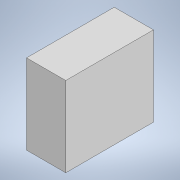
# Autodesk Inventor part: Akkuboxdummy
Saved by Autodesk Inventor 2020 (Build 240168000, 168)
## iProperties
Created: 2020-05-28
Part Number: Akkuboxdummy
Material: Generisch
Document SubType Name: Modeling
Designer: Chris
Density: 1 g/cm^3
Appearance: Vorgabe
Author: Chris
Autodesk Inventor part; units mm, degrees
ref_plane "YZ Plane" through (0, 0, 0) normal (1, 0, 0) x (0, 1, 0)
ref_plane "XZ Plane" through (0, 0, 0) normal (0, 1, 0) x (-1, 0, 0)
ref_plane "XY Plane" through (0, 0, 0) normal (0, 0, 1) x (1, 0, 0)
sketch "Skizze1" plane through (0, 0, 0) normal (0, 1, 0) x (-1, 0, 0)
  line L0 (0, 0) -> (-152, 0)
  line L1 (-152, 0) -> (-152, -340)
  line L2 (-152, -340) -> (0, -340)
  line L3 (0, -340) -> (0, 0)
  dimension "d0" = 152
  dimension "d1" = 340
  constraints: 8 end point, 2 parallel, 1 horizontal, 1 perpendicular
  measures "d0" distance of L2.end L1.end
  measures "d1" distance of L1.end L0.end
extrude "Extrusion1" add sketch "Skizze1" along normal blind 310
